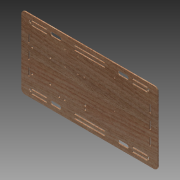
# Autodesk Inventor part: plaat
Saved by Autodesk Inventor 2015 (Build 190159000, 159)
## iProperties
Created: 2015-12-19
Part Number: plaat
Material: Generic
Document SubType Name: Modeling
Designer: david
Density: 1 g/cm^3
Appearance: Birch - Natural Polished
Author: david
Autodesk Inventor part; units mm, degrees
ref_plane "YZ Plane" through (0, 0, 0) normal (1, 0, 0) x (0, 1, 0)
ref_plane "XZ Plane" through (0, 0, 0) normal (0, 1, 0) x (-1, 0, 0)
ref_plane "XY Plane" through (0, 0, 0) normal (0, 0, 1) x (1, 0, 0)
sketch "Sketch1" plane through (0, 0, 0) normal (0, 1, 0) x (-1, 0, 0)
  line L0 (-190, 100) -> (190, 100)
  line L1 (190, 100) -> (190, -100)
  line L2 (190, -100) -> (-190, -100)
  line L3 (-190, -100) -> (-190, 100)
  line L4 (-190, 100) -> (190, -100) construction
  line L5 (190, 100) -> (-190, -100) construction
  point P0 (0, 0)
  dimension "d0" = 380
  dimension "d1" = 200
  constraints: 12 end point, 2 midpoint, 2 parallel, 1 horizontal, 1 perpendicular
  measures "d0" distance of L1.end L2.end
  measures "d1" distance of L0.end L1.end
extrude "Extrusion1" add sketch "Sketch1" along normal blind 3
sketch "Sketch3" plane through (0, 3, 0) normal (0, 1, 0) x (1, 0, 0)
  line L0 (42.5, 90.125) -> (0, 90.125)
  line L1 (0, 90.125) -> (0, 86.125)
  line L2 (0, 86.125) -> (42.5, 86.125)
  line L3 (42.5, 86.125) -> (42.5, 90.125)
  line L4 (42.5, 90.125) -> (0, 86.125) construction
  line L5 (0, 90.125) -> (42.5, 86.125) construction
  line L6 (0, 90.125) -> (-42.5, 90.125)
  line L7 (-42.5, 90.125) -> (-42.5, 86.125)
  line L8 (-42.5, 86.125) -> (0, 86.125)
  line L9 (0, 86.125) -> (0, 90.125)
  line L10 (0, 90.125) -> (-42.5, 86.125) construction
  line L11 (-42.5, 90.125) -> (0, 86.125) construction
  line L12 (190, 100) -> (-190, 100) projected
  line L13 (161.5, 90.125) -> (119, 90.125)
  line L14 (119, 90.125) -> (119, 86.125)
  line L15 (119, 86.125) -> (161.5, 86.125)
  line L16 (161.5, 86.125) -> (161.5, 90.125)
  line L17 (161.5, 90.125) -> (119, 86.125) construction
  line L18 (119, 90.125) -> (161.5, 86.125) construction
  line L19 (0, 90.125) -> (0, 90.125)
  line L20 (0, 90.125) -> (0, 86.125)
  line L21 (0, 86.125) -> (0, 86.125)
  line L22 (0, 86.125) -> (0, 90.125)
  line L23 (-119, 90.125) -> (-161.5, 90.125)
  line L24 (-161.5, 90.125) -> (-161.5, 86.125)
  line L25 (-161.5, 86.125) -> (-119, 86.125)
  line L26 (-119, 86.125) -> (-119, 90.125)
  line L27 (190, 100) -> (190, -100)
  line L28 (42.5, 79.125) -> (0, 79.125)
  line L29 (0, 79.125) -> (0, 75.125)
  line L30 (0, 75.125) -> (42.5, 75.125)
  line L31 (42.5, 75.125) -> (42.5, 79.125)
  line L32 (42.5, 79.125) -> (0, 75.125) construction
  line L33 (0, 79.125) -> (42.5, 75.125) construction
  line L34 (0, 79.125) -> (-42.5, 79.125)
  line L35 (-42.5, 79.125) -> (-42.5, 75.125)
  line L36 (-42.5, 75.125) -> (0, 75.125)
  line L37 (0, 75.125) -> (0, 79.125)
  line L38 (0, 79.125) -> (-42.5, 75.125) construction
  line L39 (-42.5, 79.125) -> (0, 75.125) construction
  line L40 (0, 79.125) -> (0, 79.125)
  line L41 (0, 79.125) -> (0, 75.125)
  line L42 (0, 75.125) -> (0, 75.125)
  line L43 (0, 75.125) -> (0, 79.125)
  line L44 (-119, 79.125) -> (-161.5, 79.125)
  line L45 (-161.5, 79.125) -> (-161.5, 75.125)
  line L46 (-161.5, 75.125) -> (-119, 75.125)
  line L47 (-119, 75.125) -> (-119, 79.125)
  line L48 (190, 89) -> (190, -111)
  line L49 (253.2147, 0) -> (-252.6779, 0)
  line L50 (161.5, 79.125) -> (119, 79.125)
  line L51 (119, 79.125) -> (119, 75.125)
  line L52 (119, 75.125) -> (161.5, 75.125)
  line L53 (161.5, 75.125) -> (161.5, 79.125)
  line L54 (161.5, 79.125) -> (119, 75.125) construction
  line L55 (119, 79.125) -> (161.5, 75.125) construction
  line L56 (42.5, -90.125) -> (0, -90.125)
  line L57 (0, -90.125) -> (0, -86.125)
  line L58 (0, -86.125) -> (42.5, -86.125)
  line L59 (42.5, -86.125) -> (42.5, -90.125)
  line L60 (42.5, -90.125) -> (0, -86.125) construction
  line L61 (0, -90.125) -> (42.5, -86.125) construction
  line L62 (0, -90.125) -> (-42.5, -90.125)
  line L63 (-42.5, -90.125) -> (-42.5, -86.125)
  line L64 (-42.5, -86.125) -> (0, -86.125)
  line L65 (0, -86.125) -> (0, -90.125)
  line L66 (0, -90.125) -> (-42.5, -86.125) construction
  line L67 (-42.5, -90.125) -> (0, -86.125) construction
  line L68 (190, -100) -> (-190, -100)
  line L69 (161.5, -90.125) -> (119, -90.125)
  line L70 (119, -90.125) -> (119, -86.125)
  line L71 (119, -86.125) -> (161.5, -86.125)
  line L72 (161.5, -86.125) -> (161.5, -90.125)
  line L73 (161.5, -90.125) -> (119, -86.125) construction
  line L74 (119, -90.125) -> (161.5, -86.125) construction
  line L75 (0, -90.125) -> (0, -90.125)
  line L76 (0, -90.125) -> (0, -86.125)
  line L77 (0, -86.125) -> (0, -86.125)
  line L78 (0, -86.125) -> (0, -90.125)
  line L79 (-119, -90.125) -> (-161.5, -90.125)
  line L80 (-161.5, -90.125) -> (-161.5, -86.125)
  line L81 (-161.5, -86.125) -> (-119, -86.125)
  line L82 (-119, -86.125) -> (-119, -90.125)
  line L83 (0, -79.125) -> (0, -79.125)
  line L84 (0, -75.125) -> (0, -75.125)
  line L85 (0, -75.125) -> (0, -79.125)
  line L86 (0, -79.125) -> (0, -75.125)
  line L87 (-42.5, -75.125) -> (0, -75.125)
  line L88 (-42.5, -79.125) -> (-42.5, -75.125)
  line L89 (0, -79.125) -> (-42.5, -75.125) construction
  line L90 (-42.5, -79.125) -> (0, -75.125) construction
  line L91 (0, -79.125) -> (-42.5, -79.125)
  line L92 (0, -79.125) -> (0, -75.125)
  line L93 (0, -75.125) -> (0, -79.125)
  line L94 (42.5, -79.125) -> (0, -79.125)
  line L95 (0, -75.125) -> (42.5, -75.125)
  line L96 (42.5, -79.125) -> (0, -75.125) construction
  line L97 (0, -79.125) -> (42.5, -75.125) construction
  line L98 (42.5, -75.125) -> (42.5, -79.125)
  line L99 (-119, -75.125) -> (-119, -79.125)
  line L100 (-119, -79.125) -> (-161.5, -79.125)
  line L101 (-161.5, -75.125) -> (-119, -75.125)
  line L102 (-161.5, -79.125) -> (-161.5, -75.125)
  line L103 (119, -79.125) -> (119, -75.125)
  line L104 (161.5, -79.125) -> (119, -79.125)
  line L105 (119, -75.125) -> (161.5, -75.125)
  line L106 (161.5, -79.125) -> (119, -75.125) construction
  line L107 (119, -79.125) -> (161.5, -75.125) construction
  line L108 (161.5, -75.125) -> (161.5, -79.125)
  point P0 (0, 0)
  point P1 (21.25, 88.125)
  point P2 (-21.25, 88.125)
  point P3 (140.25, 88.125)
  point P4 (0, -11)
  point P5 (21.25, 77.125)
  point P6 (-21.25, 77.125)
  point P7 (-190, 89)
  point P8 (140.25, 77.125)
  point P9 (21.25, -88.125)
  point P10 (-21.25, -88.125)
  point P11 (140.25, -88.125)
  point P12 (190, -89)
  point P13 (-190, -89)
  point P14 (-21.25, -77.125)
  point P15 (21.25, -77.125)
  point P16 (140.25, -77.125)
  dimension "d49" = 10
  dimension "d28" = 42.5
  dimension "d29" = 4
  dimension "d30" = 42.5
  dimension "d31" = 4
  dimension "d32" = 0
  dimension "d33" = 0
  dimension "d34" = 9.875
  dimension "d35" = 9.875
  dimension "d36" = 42.5
  dimension "d37" = 4
  dimension "d38" = 76.5
  dimension "d39" = 9.875
  dimension "d40" = 42.5
  dimension "d41" = 4
  dimension "d42" = 76.5
  dimension "d43" = 9.875
  dimension "d46" = 11
  dimension "d53" = 11
  dimension "d68" = 71
  dimension "d69" = 100
  constraints: 216 end point, 45 symmetric about line, 24 midpoint, 10 equal length, 6 horizontal, 5 perpendicular, 3 vertical, 1 collinear, 51 other
  measures "d28" distance of L2.end L1.end
  measures "d29" distance of L1.end L0.end
  measures "d30" distance of L8.end L7.end
  measures "d31" distance of L7.end L6.end
  measures "d32" distance from line of L9 point (0, 0)
  measures "d33" distance between parallel lines of L1 L9
  measures "d34" distance between parallel lines of L12 L6
  measures "d35" distance between parallel lines of L12 L0
  measures "d36" distance of L15.end L14.end
  measures "d37" distance of L14.end L13.end
  measures "d38" distance of L0.start L13.end
  measures "d39" distance between parallel lines of L12 L13
  measures "d40" distance of L25.end L24.end
  measures "d41" distance of L24.end L23.end
  measures "d42" horizontal distance of L7.end L23.start
  measures "d43" distance between parallel lines of L12 L23
  measures "d46" distance of point (0, 0) point (0, -11)
  measures "d53" distance of L14.end L51.end
  measures "d68" distance between parallel lines of L14 L27
  measures "d69" distance between parallel lines of L12 L49
extrude "Extrusion3" cut sketch "Sketch3" against normal blind 10
sketch "Sketch4" plane through (0, 3, 0) normal (0, 1, 0) x (1, 0, 0)
  line L0 (170.5, 29) -> (166.5, 29)
  line L1 (166.5, 29) -> (166.5, 51)
  line L2 (166.5, 51) -> (170.5, 51)
  line L3 (170.5, 51) -> (170.5, 29)
  line L4 (170.5, 29) -> (166.5, 51) construction
  line L5 (166.5, 29) -> (170.5, 51) construction
  line L6 (-167.5, 29) -> (-171.5, 29)
  line L7 (-171.5, 29) -> (-171.5, 51)
  line L8 (-171.5, 51) -> (-167.5, 51)
  line L9 (-167.5, 51) -> (-167.5, 29)
  line L10 (-167.5, 29) -> (-171.5, 51) construction
  line L11 (-171.5, 29) -> (-167.5, 51) construction
  line L12 (190, 100) -> (190, -100) projected
  line L13 (-190, 100) -> (-190, -100) projected
  line L14 (190, 100) -> (-190, 100) projected
  point P0 (0, 0)
  point P1 (168.5, 40)
  point P2 (-169.5, 40)
  dimension "d60" = 4
  dimension "d61" = 22
  dimension "d62" = 4
  dimension "d63" = 22
  dimension "d64" = 19.5
  dimension "d65" = 18.5
  dimension "d93" = 49
  dimension "d94" = 49
  constraints: 24 end point, 4 midpoint, 4 parallel, 2 horizontal, 2 perpendicular
  measures "d60" distance of L1.end L2.end
  measures "d61" distance of L0.end L1.end
  measures "d62" distance of L7.end L8.end
  measures "d63" distance of L6.end L7.end
  measures "d64" distance between parallel lines of L12 L3
  measures "d65" distance between parallel lines of L13 L7
  measures "d93" distance between parallel lines of L14 L2
  measures "d94" distance between parallel lines of L14 L8
extrude "Extrusion4" cut sketch "Sketch4" against normal blind 10
sketch "Sketch5" plane through (0, 3, 0) normal (0, 1, 0) x (1, 0, 0)
  line L0 (-162.5, -26.6595) -> (-157.5, -26.6595)
  line L1 (-157.5, -26.6595) -> (-157.5, -21.6595)
  line L2 (-157.5, -21.6595) -> (-162.5, -21.6595)
  line L3 (-162.5, -21.6595) -> (-162.5, -26.6595)
  line L4 (-162.5, 37.4377) -> (-157.5, 37.4377)
  line L5 (-157.5, 37.4377) -> (-157.5, 42.4377)
  line L6 (-157.5, 42.4377) -> (-162.5, 42.4377)
  line L7 (-162.5, 42.4377) -> (-162.5, 37.4377)
  line L8 (-112.5, 37.4377) -> (-107.5, 37.4377)
  line L9 (-107.5, 37.4377) -> (-107.5, 42.4377)
  line L10 (-107.5, 42.4377) -> (-112.5, 42.4377)
  line L11 (-112.5, 42.4377) -> (-112.5, 37.4377)
  line L12 (-112.5, -21.6595) -> (-107.5, -21.6595)
  line L13 (-107.5, -21.6595) -> (-107.5, -26.6595)
  line L14 (-107.5, -26.6595) -> (-112.5, -26.6595)
  line L15 (-112.5, -26.6595) -> (-112.5, -21.6595)
  line L16 (-167.5, 51) -> (-167.5, 29) projected
  point P0 (0, 0)
  dimension "d72" = 5
  dimension "d73" = 5
  dimension "d74" = 5
  dimension "d75" = 5
  dimension "d76" = 5
  dimension "d77" = 5
  dimension "d78" = 5
  dimension "d79" = 45
  dimension "d80" = 45
  constraints: 32 end point, 8 parallel, 6 point on line, 4 horizontal, 4 perpendicular
  measures "d72" distance of L2.end L1.end
  measures "d73" distance of L1.end L0.end
  measures "d74" distance of L6.end L5.end
  measures "d75" distance of L5.end L4.end
  measures "d76" distance of L10.end L9.end
  measures "d77" distance of L9.end L8.end
  measures "d78" distance between parallel lines of L16 L3
  measures "d79" distance between parallel lines of L1 L15
  measures "d80" distance between parallel lines of L11 L5
extrude "Extrusion5" cut sketch "Sketch5" against normal blind 10
sketch "Sketch6" plane through (0, 3, 0) normal (0, 1, 0) x (1, 0, 0)
  line L0 (-87.5, 60.125) -> (-82.5, 60.125)
  line L1 (-82.5, 60.125) -> (-82.5, 55.125)
  line L2 (-82.5, 55.125) -> (-87.5, 55.125)
  line L3 (-87.5, 55.125) -> (-87.5, 60.125)
  line L4 (-72.5, 60.125) -> (-67.5, 60.125)
  line L5 (-67.5, 60.125) -> (-67.5, 55.125)
  line L6 (-67.5, 55.125) -> (-72.5, 55.125)
  line L7 (-72.5, 55.125) -> (-72.5, 60.125)
  line L8 (-107.5, 42.4377) -> (-107.5, 37.4377) projected
  line L9 (42.5, 75.125) -> (-42.5, 75.125) projected
  line L10 (-15, 45) -> (-10, 45)
  line L11 (-10, 45) -> (-10, 40)
  line L12 (-10, 40) -> (-15, 40)
  line L13 (-15, 40) -> (-15, 45)
  line L14 (-15, 45) -> (-10, 40) construction
  line L15 (-10, 45) -> (-15, 40) construction
  line L16 (-10, 55) -> (-15, 55)
  line L17 (-15, 55) -> (-15, 50)
  line L18 (-15, 50) -> (-10, 50)
  line L19 (-10, 50) -> (-10, 55)
  line L20 (-10, 55) -> (-15, 50) construction
  line L21 (-15, 55) -> (-10, 50) construction
  point P0 (0, 0)
  point P1 (-12.5, 42.5)
  point P2 (-12.5, 52.5)
  dimension "d83" = 5
  dimension "d84" = 5
  dimension "d85" = 5
  dimension "d86" = 10
  dimension "d87" = 20
  dimension "d88" = 15
  dimension "d89" = 5
  dimension "d90" = 15
  dimension "d159" = 5
  dimension "d160" = 5
  dimension "d162" = 40
  dimension "d163" = 10
  dimension "d164" = 5
  dimension "d165" = 5
  dimension "d166" = 5
  dimension "d167" = 10
  constraints: 40 end point, 8 parallel, 4 horizontal, 4 midpoint, 4 perpendicular
  measures "d83" distance of L1.end L2.end
  measures "d84" distance of L0.end L1.end
  measures "d85" distance of L5.end L6.end
  measures "d86" distance between parallel lines of L1 L7
  measures "d87" distance between parallel lines of L8 L3
  measures "d88" distance between parallel lines of L9 L4
  measures "d89" distance of L4.end L5.end
  measures "d90" distance between parallel lines of L9 L0
  measures "d159" distance of L11.end L12.end
  measures "d160" distance of L10.end L11.end
  measures "d162" distance from line of point (0, 0) L12
  measures "d163" distance from line of point (0, 0) L11
  measures "d164" distance of L18.end L17.end
  measures "d165" distance of L17.end L16.end
  measures "d166" distance between parallel lines of L10 L18
  measures "d167" distance from line of point (0, 0) L19
extrude "Extrusion6" cut sketch "Sketch6" against normal blind 10
pattern_linear "Rectangular Pattern1" count 3 spacing 40 along (0, 0, 1) of "Extrusion4"
sketch "Sketch7" plane through (0, 0, 0) normal (0, -1, 0) x (1, 0, 0)
  circle A0 centre (163, -82.5) radius 3.5
  circle A1 centre (-165, -82.5) radius 3.5
  line L0 (190, -100) -> (190, 100) projected
  line L1 (-190, 100) -> (-190, -100) projected
  line L2 (-190, -100) -> (190, -100) projected
  line L3 (190, 100) -> (190, -100) projected
  line L4 (190, 0) -> (-190, 0)
  circle A2 centre (163, 82.5) radius 3.5
  circle A3 centre (-165, 82.5) radius 3.5
  line L5 (-190, 100) -> (190, 100)
  point P0 (0, 0)
  point P1 (2.5, -82.5)
  point P2 (2.5, 82.5)
  dimension "d99" = 0
  dimension "d98" = 7
  dimension "d100" = 7
  dimension "d102" = 160.5
  dimension "d103" = 167.5
  dimension "d104" = 25
  dimension "d105" = 17.5
  dimension "d106" = 17.5
  dimension "d107" = 17.5
  dimension "d110" = 27
  constraints: 4 centre point, 4 end point, 3 symmetric about line, 2 midpoint, 1 horizontal, 6 other
  measures "d98" diameter of A0
  measures "d100" diameter of A1
  measures "d102" distance of point (2.5, -82.5) A0.centre
  measures "d103" distance of A1.centre point (2.5, -82.5)
  measures "d104" distance from line of L1 A1.centre
  measures "d105" distance from line of L2 A1.centre
  measures "d106" distance from line of L2 point (2.5, -82.5)
  measures "d107" distance from line of L2 A0.centre
  measures "d110" distance from line of L0 A0.centre
extrude "Extrusion7" cut sketch "Sketch7" against normal blind 10 contours A0 | A1 | A2 | A3
sketch "Sketch8" plane through (0, 0, 0) normal (0, -1, 0) x (1, 0, 0)
  line L0 (-104, 83) -> (-84, 83) construction
  line L1 (-104, 78) -> (-84, 78)
  line L2 (-84, 88) -> (-104, 88)
  arc A0 (-104, 88) -> (-104, 78) centre (-104, 83) ccw
  arc A1 (-84, 78) -> (-84, 88) centre (-84, 83) ccw
  line L3 (-104, 83) -> (-84, 83) construction
  line L4 (-104, -83) -> (-84, -83) construction
  line L5 (-104, -88) -> (-84, -88)
  line L6 (-84, -78) -> (-104, -78)
  arc A2 (-104, -78) -> (-104, -88) centre (-104, -83) ccw
  arc A3 (-84, -88) -> (-84, -78) centre (-84, -83) ccw
  line L7 (-190, -100) -> (190, -100) projected
  line L8 (190, 100) -> (-190, 100) projected
  line L9 (-119, -86.125) -> (-119, -90.125) projected
  line L10 (-119, 79.125) -> (-119, 75.125) projected
  line L11 (84, -83) -> (104, -83) construction
  line L12 (84, -88) -> (104, -88)
  line L13 (104, -78) -> (84, -78)
  arc A4 (84, -78) -> (84, -88) centre (84, -83) ccw
  arc A5 (104, -88) -> (104, -78) centre (104, -83) ccw
  line L14 (84, -83) -> (104, -83) construction
  line L15 (119, -90.125) -> (119, -86.125) projected
  line L16 (104, 83) -> (84, 83) construction
  line L17 (104, 88) -> (84, 88)
  line L18 (84, 78) -> (104, 78)
  arc A6 (104, 78) -> (104, 88) centre (104, 83) ccw
  arc A7 (84, 88) -> (84, 78) centre (84, 83) ccw
  line L19 (119, 86.125) -> (119, 90.125) projected
  point P0 (0, 0)
  point P1 (-94, 83)
  point P2 (-94, -83)
  point P3 (94, -83)
  point P4 (94, 83)
  dimension "d111" = 20
  dimension "d112" = 0
  dimension "d113" = 10
  dimension "d114" = 20
  dimension "d115" = 10
  dimension "d116" = 12
  dimension "d117" = 12
  dimension "d118" = 15
  dimension "d119" = 15
  dimension "d120" = 20
  dimension "d121" = 0
  dimension "d122" = 10
  dimension "d123" = 12
  dimension "d124" = 15
  dimension "d125" = 20
  dimension "d126" = 10
  dimension "d127" = 12
  dimension "d128" = 15
  constraints: 36 end point, 16 point on circle, 16 tangent, 8 centre point, 5 horizontal, 5 parallel, 4 midpoint, 2 collinear
  measures "d111" distance of L0.start L0.end
  measures "d112" distance between parallel lines of L0 L3
  measures "d113" diameter of A1
  measures "d114" distance of L4.start L4.end
  measures "d115" diameter of A3
  measures "d116" distance between parallel lines of L7 L5
  measures "d117" distance between parallel lines of L8 L2
  measures "d118" distance from line of L9 L4.start
  measures "d119" distance from line of L10 L0.start
  measures "d120" distance of L11.start L11.end
  measures "d121" distance between parallel lines of L11 L14
  measures "d122" diameter of A5
  measures "d123" distance between parallel lines of L7 L12
  measures "d124" distance from line of L15 L11.end
  measures "d125" distance of L16.start L16.end
  measures "d126" diameter of A7
  measures "d127" distance between parallel lines of L8 L17
  measures "d128" distance from line of L19 L16.start
extrude "Extrusion8" cut sketch "Sketch8" against normal blind 10
fillet "Fillet1" radius 10 4 edges at (-190, 1.5, 100) (190, 1.5, 100) (190, 1.5, -100) (-190, 1.5, -100)
sketch "Sketch9" plane through (0, 3, 0) normal (0, 1, 0) x (1, 0, 0)
  circle A0 centre (-32.5, -65) radius 1.75
  circle A1 centre (-32.5, -22.5) radius 1.75
  circle A2 centre (-68.5, -22.5) radius 1.75
  circle A3 centre (-68.5, -65) radius 1.75
  line L0 (-180, -100) -> (180, -100) projected
  line L1 (-42.5, -79.125) -> (-42.5, -75.125) projected
  point P0 (0, 0)
  dimension "d132" = 3.5
  dimension "d133" = 3.5
  dimension "d134" = 3.5
  dimension "d135" = 3.5
  dimension "d136" = 36
  dimension "d137" = 36
  dimension "d138" = 42.5
  dimension "d139" = 42.5
  dimension "d140" = 35
  dimension "d141" = 35
  dimension "d142" = 36
  dimension "d143" = 10
  constraints: 4 centre point
  measures "d132" diameter of A0
  measures "d133" diameter of A1
  measures "d134" diameter of A2
  measures "d135" diameter of A3
  measures "d136" distance of A0.centre A3.centre
  measures "d137" distance of A2.centre A1.centre
  measures "d138" distance of A2.centre A3.centre
  measures "d139" distance of A1.centre A0.centre
  measures "d140" distance from line of L0 A3.centre
  measures "d141" distance from line of L0 A0.centre
  measures "d142" horizontal distance of A1.centre A3.centre
  measures "d143" distance from line of L1 A0.centre
extrude "Extrusion9" cut sketch "Sketch9" against normal blind 10
sketch "Sketch10" plane through (0, 3, 0) normal (0, 1, 0) x (1, 0, 0)
  circle A0 centre (70, 15) radius 1.75
  circle A1 centre (-15, -25) radius 1.75
  circle A2 centre (70, -65) radius 1.75
  point P0 (0, 0)
  dimension "d146" = 3.5
  dimension "d147" = 3.5
  dimension "d148" = 3.5
  dimension "d149" = 70
  dimension "d150" = 15
  dimension "d151" = 25
  dimension "d152" = 65
  dimension "d153" = 15
  dimension "d154" = 70
  constraints: 3 centre point
  measures "d146" diameter of A0
  measures "d147" diameter of A1
  measures "d148" diameter of A2
  measures "d149" horizontal distance of A0.centre point (0, 0)
  measures "d150" horizontal distance of A1.centre point (0, 0)
  measures "d151" vertical distance of A1.centre point (0, 0)
  measures "d152" vertical distance of point (0, 0) A2.centre
  measures "d153" vertical distance of point (0, 0) A0.centre
  measures "d154" horizontal distance of A2.centre point (0, 0)
extrude "Extrusion10" cut sketch "Sketch10" against normal blind 10
body "Solid1" dims "d125" = 20, "d126" = 10, "d127" = 12, "d128" = 15
